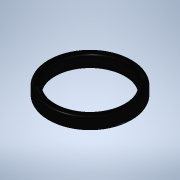
# Autodesk Inventor part: YTP-AP-E20-R1.0
Saved by Autodesk Inventor 2020.4 (Build 244396000, 396)
## iProperties
RuleStatus: InUse
AfterDocNew0: iPropertyEnforcement
BeforeDocSave0: Materialprüfung
Created: 2021-08-29
Part Number: YTP-AP-E20-R1.0
Material: Gummi, Silikon
Document SubType Name: Modeling
Designer: Uwe Wieser
Mass: 0.0139752 g
Surface Area: 0.550171 cm^2
Volume: 0.0111801 cm^3
Density: 1.25 g/cm^3
Appearance: Schwarz
Project: Airbrush
Description: Dichtring-Ventil
Werkstoff: Gummi
Author: Uwe Wieser
Autodesk Inventor part; units mm, degrees
ref_plane "YZ Plane" through (0, 0, 0) normal (1, 0, 0) x (0, 1, 0)
ref_plane "XZ Plane" through (0, 0, 0) normal (0, 1, 0) x (-1, 0, 0)
ref_plane "XY Plane" through (0, 0, 0) normal (0, 0, 1) x (1, 0, 0)
sketch "Skizze1" plane through (0, 0, 0) normal (0, 0, 1) x (1, 0, 0)
  circle A0 centre (0, 0) radius 2.7
  circle A1 centre (0, 0) radius 3.325
  dimension "d0" = 5.4
  dimension "d1" = 6.65
  constraints: 2 centre point, 2 coincident
  measures "d0" diameter of A0
  measures "d1" diameter of A1
extrude "Extrusion1" add sketch "Skizze1" along normal mid plane 1
fillet "Rundung1" radius 0.2 4 edges at (-3.325, 0, 0.5) (-3.325, 0, -0.5) (-2.7, 0, 0.5) (-2.7, 0, -0.5)
